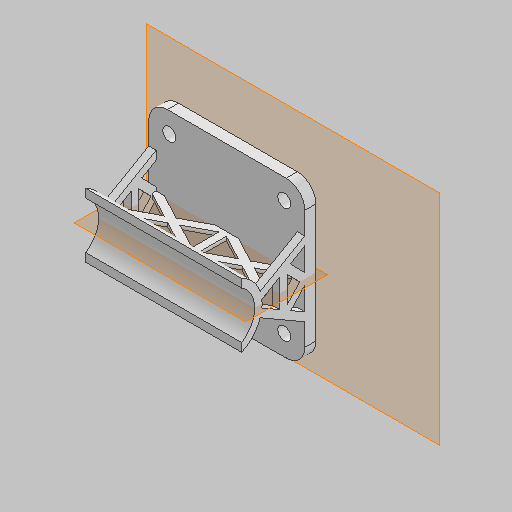
# Autodesk Inventor part: Arnes cable EJE z
Saved by Autodesk Inventor 2025.3 (Build 293356000, 356)
## iProperties
Created: 2025-11-14
Part Number: Arnes cable EJE z
Material: Genérico
Document SubType Name: Modeling
Designer: Inema
Density: 1 g/cm^3
Appearance: Valor por defecto
Author: Inema
Autodesk Inventor part; units mm, degrees
ref_plane "YZ Plane" through (0, 0, 0) normal (1, 0, 0) x (0, 1, 0)
ref_plane "XZ Plane" through (0, 0, 0) normal (0, 1, 0) x (-1, 0, 0)
ref_plane "XY Plane" through (0, 0, 0) normal (0, 0, 1) x (1, 0, 0)
ref_plane "Plano de trabajo1" through (0, 0, 0) normal (0, 0, 1) x (1, 0, 0)
sketch "Boceto1" plane through (0, 0, 0) normal (0, 0, 1) x (1, 0, 0)
  circle A0 centre (-91.78, -12) radius 1.75 projected
  circle A1 centre (-60.78, -12) radius 1.75 projected
  circle A2 centre (-60.78, -43) radius 1.75 projected
  circle A3 centre (-91.78, -43) radius 1.75 projected
  line L0 (-92.28, -48.5) -> (-55.1363, -48.5) projected
  line L1 (-55.28, -6.5435) -> (-97.28, -6.5435)
  line L2 (-97.28, -6.5435) -> (-97.28, -48.5)
  line L3 (-97.28, -48.5) -> (-55.28, -48.5)
  line L4 (-55.28, -48.5) -> (-55.28, -6.5435)
  point P0 (0, 0)
  point P1 (-55.28, -48.5)
  dimension "d0" = 5.5
  dimension "d1" = 5.5
  dimension "d2" = 5.5
  dimension "d3" = 5.4565
  constraints: 8 end point, 2 parallel, 1 horizontal, 1 perpendicular
  measures "d0" distance from line of A3.centre L3
  measures "d1" distance from line of A3.centre L2
  measures "d2" distance from line of A2.centre L4
  measures "d3" distance from line of A1.centre L1
extrude "Extrusión1" add sketch "Boceto1" along normal blind 3
fillet "Empalme1" radius 5 4 edges at (-55.28, -6.5435, 1.5) (-97.28, -6.5435, 1.5) (-97.28, -48.5, 1.5) (-55.28, -48.5, 1.5)
sketch "Boceto2" plane through (-97.28, -48.5, 0) normal (-1, 0, 0) x (0, 0, 1)
  arc A0 (20, 27.3226) -> (20, 14.634) centre (24, 20.9783) ccw
  line L0 (0, 58.2) -> (0, -9.7) projected
  line L1 (3, 36.9565) -> (3, 5) projected
  arc A1 (20, 29.5951) -> (20, 12.3614) centre (24, 20.9783) ccw
  line L2 (20, 29.5951) -> (20, 27.3226)
  line L3 (20, 14.634) -> (20, 12.3614)
  point P0 (0, 48.5)
  point P1 (3, 20.9783)
  dimension "d7" = 15
  dimension "d8" = 24
  dimension "d9" = 2
  dimension "d11" = 17
  constraints: 4 end point, 4 point on circle, 2 centre point, 2 vertical, 1 horizontal alignment, 1 midpoint
  measures "d7" diameter of A0
  measures "d8" distance from line of A0.centre L0
  measures "d9" radial gap between concentric circles of A0 A1
  measures "d11" distance from line of L3.end L1
extrude "Extrusión2" add sketch "Boceto2" against normal up to surface (42 mm away)
sketch "Boceto3" plane through (-97.28, -43.5, 0) normal (-1, 0, 0) x (0, 0, 1)
  arc A0 (20, 24.5951) -> (20, 7.3614) centre (24, 15.9783) ccw projected
  line L0 (15.0086, 19.0451) -> (3, 25.9783)
  line L1 (3, 0) -> (3, 31.9565) projected
  line L2 (15.0086, 12.9115) -> (3, 5.9783)
  line L3 (3, 23.6689) -> (14.5549, 16.9977)
  line L4 (14.5549, 14.9589) -> (3, 8.2877)
  line L5 (8.7774, 20.3333) -> (8.7774, 11.6233) construction
  line L6 (9.7774, 19.7559) -> (9.7774, 12.2006)
  line L7 (7.7774, 20.9106) -> (7.7774, 11.0459)
  line L8 (7.7774, 20.9106) -> (3, 15.9783) construction
  line L9 (7.6379, 10.9654) -> (3, 15.9783) construction
  line L10 (7.7774, 12.2871) -> (4.3769, 15.9625)
  line L11 (6.7499, 10.4527) -> (3, 14.5058)
  line L12 (7.7774, 19.4733) -> (4.3769, 15.9625)
  line L13 (6.8846, 21.4261) -> (3, 17.4156)
  line L14 (14.5, 15.9783) -> (13.0426, 15.9783) construction
  arc A1 (20, 24.5951) -> (20, 7.3614) centre (24, 15.9783) ccw construction
  point P0 (0, 43.5)
  point P1 (9.7774, 15.9783)
  point P2 (14.5, 15.9783)
  dimension "d14" = 20
  dimension "d15" = 2
  dimension "d16" = 1
  dimension "d17" = 1
  dimension "d18" = 1
  dimension "d19" = 1
  dimension "d20" = 1
  dimension "d21" = 1
  dimension "d22" = 2
  dimension "d23" = 60
  dimension "d24" = 30
  constraints: 28 end point, 9 point on line, 6 parallel, 6 point on circle, 3 midpoint, 1 horizontal, 1 horizontal alignment, 8 other
  measures "d14" distance of L2.end L0.end
  measures "d15" distance between parallel lines of L0 L3
  measures "d16" distance between parallel lines of L5 L6
  measures "d17" distance between parallel lines of L7 L5
  measures "d18" distance between parallel lines of L9 L10
  measures "d19" distance between parallel lines of L12 L8
  measures "d20" distance between parallel lines of L8 L13
  measures "d21" distance between parallel lines of L11 L9
  measures "d22" distance between parallel lines of L2 L4
  measures "d23" angle of L4 L3
  measures "d24" angle of L4 L14
extrude "Extrusión3" add sketch "Boceto3" against normal blind 2 contours A0 L3 L1 L0 | A0 L2 L1 L4 | L6 L4 L7 L3 | L7 L12 L10 L4 L11 L1 L13 L3
sketch "Boceto4" plane through (-55.28, -27.5217, 24) normal (1, 0, 0) x (0, 0, -1)
  line L0 (21, 1.4373) -> (17.1154, 5.4479) projected
  line L1 (17.1154, 5.4479) -> (21, 7.6906) projected
  line L2 (21, 10) -> (21, 7.6906) projected
  line L3 (21, 10) -> (8.9914, 3.0668) projected
  arc A0 (9.4451, 1.0194) -> (8.9914, 3.0668) centre (0, 0) ccw projected
  line L4 (9.4451, 1.0194) -> (14.2226, 3.7777) projected
  line L5 (14.2226, 3.7777) -> (14.2226, -3.7777) projected
  line L6 (14.2226, -3.7777) -> (9.4451, -1.0194) projected
  arc A1 (8.9914, -3.0668) -> (9.4451, -1.0194) centre (0, 0) ccw projected
  line L7 (8.9914, -3.0668) -> (21, -10) projected
  line L8 (21, -7.6906) -> (21, -10) projected
  line L9 (21, -7.6906) -> (17.2501, -5.5256) projected
  line L10 (17.2501, -5.5256) -> (21, -1.4725) projected
  line L11 (21, 1.4373) -> (21, -1.4725) projected
  line L12 (16.2226, -3.6912) -> (16.2226, 3.495) projected
  line L13 (16.2226, 3.495) -> (19.6231, -0.0158) projected
  line L14 (19.6231, -0.0158) -> (16.2226, -3.6912) projected
  point P0 (24, 27.5217)
extrude "Extrusión4" add sketch "Boceto4" against normal blind 2
ref_plane "Plano de trabajo2" through (-92.28, -27.5217, 0) normal (0, 1, 0) x (1, 0, 0)
sketch "Boceto5" plane through (-92.28, -27.5217, 0) normal (0, 1, 0) x (1, 0, 0)
  line L0 (-3, -14.5) -> (35, -14.5)
  line L1 (35, -14.5) -> (35, -12.5)
  line L2 (35, -12.5) -> (-3, -12.5)
  line L3 (-3, -12.5) -> (-3, -14.5)
  line L4 (-5, -14.5) -> (37, -14.5) projected
  line L5 (-3, -15.0086) -> (-3, -3) projected
  line L6 (35, -3) -> (35, -15.0086) projected
  line L7 (16, -12.5) -> (16, -3) construction
  line L8 (0, -3) -> (32, -3) construction
  line L9 (15, -12.5) -> (15, -3)
  line L10 (17, -12.5) -> (17, -3)
  line L11 (17, -3) -> (35, -12.5) construction
  line L12 (37, -3) -> (35, -3) projected
  line L13 (17, -12.5) -> (35, -3) construction
  line L14 (-3, -12.5) -> (15, -3) construction
  line L15 (15, -12.5) -> (-3, -3) construction
  line L16 (12.8576, -12.5) -> (-3, -4.1307)
  line L17 (15, -11.3693) -> (-0.8576, -3)
  line L18 (-0.8576, -12.5) -> (15, -4.1307)
  line L19 (-3, -11.3693) -> (12.8576, -3)
  line L20 (19.1424, -12.5) -> (35, -4.1307)
  line L21 (17, -11.3693) -> (32.8576, -3)
  line L22 (17, -4.1307) -> (32.8576, -12.5)
  line L23 (19.1424, -3) -> (35, -11.3693)
  line L24 (2.25, -3) -> (-1.25, -3) projected
  line L25 (33.25, -3) -> (29.75, -3) projected
  line L26 (33.25, -3) -> (29.75, -3) projected
  line L27 (2.25, -3) -> (-1.25, -3) projected
  line L28 (37, -3) -> (35, -3) projected
  line L29 (35, -3) -> (37, -3) projected
  line L30 (37, -3) -> (35, -3) projected
  line L31 (35, -3) -> (37, -3) projected
  line L32 (32, -3) -> (37, -3) projected
  line L33 (32, -3) -> (0, -3) projected
  line L34 (-5, -3) -> (0, -3) projected
  line L35 (-5, -3) -> (-3, -3) projected
  line L36 (-3, -3) -> (-5, -3) projected
  line L37 (-5, -3) -> (-3, -3) projected
  line L38 (-3, -3) -> (-5, -3) projected
  line L39 (-5, -3) -> (-3, -3) projected
  line L40 (-3, -3) -> (-5, -3) projected
  line L41 (0, -3) -> (-5, -3) projected
  line L42 (0, -3) -> (32, -3) projected
  line L43 (37, -3) -> (32, -3) projected
  line L44 (37, -3) -> (35, -3) projected
  line L45 (35, -3) -> (37, -3) projected
  point P0 (92.28, 0)
  point P1 (6, -8.8807)
  point P2 (8.1424, -7.75)
  point P3 (23.8576, -7.75)
  point P4 (26, -8.8807)
  point P5 (28.1424, -7.75)
  point P6 (26, -6.6193)
  point P7 (19.1424, -3)
  point P8 (6, -6.6193)
  point P9 (-0.8576, -3)
  point P10 (3.8576, -7.75)
  dimension "d29" = 2
  dimension "d30" = 1
  dimension "d31" = 1
  dimension "d32" = 1
  dimension "d33" = 1
  dimension "d34" = 1
  dimension "d35" = 1
  dimension "d36" = 1
  dimension "d37" = 1
  dimension "d38" = 1
  dimension "d39" = 1
  constraints: 38 end point, 16 point on line, 12 parallel, 3 collinear, 2 midpoint, 1 horizontal, 1 perpendicular
  measures "d29" distance of L1.end L0.end
  measures "d30" distance between parallel lines of L7 L9
  measures "d31" distance between parallel lines of L7 L10
  measures "d32" distance between parallel lines of L15 L16
  measures "d33" distance between parallel lines of L15 L17
  measures "d34" distance between parallel lines of L14 L19
  measures "d35" distance between parallel lines of L14 L18
  measures "d36" distance between parallel lines of L13 L20
  measures "d37" distance between parallel lines of L13 L21
  measures "d38" distance between parallel lines of L11 L22
  measures "d39" distance between parallel lines of L11 L23
extrude "Extrusión5" add sketch "Boceto5" along normal mid plane 1 contours L3 L2 L1 L0 | L5 L19 L16 L18 L2 | L2 L22 L20 L23 L6 | L16 L18 L17 L9 L2 | L16 L19 L17 L18 | L5 L34 L24 L17 L19 L16 | L2 L10 L21 L22 L20 | L22 L21 L23 L20 | L20 L23 L21 L25 L32 L6 | L9 L33 L10 L2 | L17 L19 L33 L9 L18 | L22 L10 L33 L23 L21
sketch "Boceto6" plane through (-92.28, -28.0217, 0) normal (0, -1, 0) x (1, 0, 0)
  line L0 (3.5, 14) -> (8.5, 14)
  line L1 (8.5, 14) -> (8.5, 13)
  line L2 (8.5, 13) -> (3.5, 13)
  line L3 (3.5, 13) -> (3.5, 14)
  line L4 (23.5, 14) -> (28.5, 14)
  line L5 (28.5, 14) -> (28.5, 13)
  line L6 (28.5, 13) -> (23.5, 13)
  line L7 (23.5, 13) -> (23.5, 14)
  line L8 (19.1424, 12.5) -> (32.8576, 12.5) projected
  line L9 (-0.8576, 12.5) -> (12.8576, 12.5) projected
  point P0 (92.28, 0)
  point P1 (6, 13)
  point P2 (6, 12.5)
  point P3 (26, 13)
  point P4 (26, 12.5)
  dimension "d42" = 1
  dimension "d43" = 0.5
  dimension "d44" = 5
  constraints: 16 end point, 4 midpoint, 4 parallel, 2 equal length, 2 horizontal, 2 perpendicular, 2 vertical alignment, 1 point on line
  measures "d42" distance of L4.end L5.end
  measures "d43" distance between parallel lines of L8 L6
  measures "d44" distance of L5.end L6.end
extrude "Extrusión6" cut sketch "Boceto6" against normal blind 1
equation "\"d2\" = d1"
equation "\"d24\" = 0.5 * d23"
equation "\"d35\" = d34"
